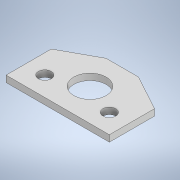
# Autodesk Inventor part: PositioningStop
Saved by Autodesk Inventor 2022.2 (Build 262287030, 287C)
## iProperties
Created: 2023-02-06
Part Number: PositioningStop
Material: Generic
Document SubType Name: Modeling
Designer: jak27277
Density: 1 g/cm^3
Appearance: Default
Author: jak27277
Autodesk Inventor part; units mm, degrees
ref_plane "YZ Plane" through (0, 0, 0) normal (1, 0, 0) x (0, 1, 0)
ref_plane "XZ Plane" through (0, 0, 0) normal (0, 1, 0) x (-1, 0, 0)
ref_plane "XY Plane" through (0, 0, 0) normal (0, 0, 1) x (1, 0, 0)
sketch "Sketch1" plane through (0, 0, 0) normal (0, 1, 0) x (-1, 0, 0)
  circle A0 centre (0, 0) radius 15.875
  line L0 (0, -31.75) -> (15.875, -31.75)
  line L1 (15.875, -31.75) -> (50.8, -12.7)
  line L2 (50.8, -12.7) -> (50.8, 31.75)
  line L3 (50.8, 31.75) -> (0, 31.75)
  circle A1 centre (31.75, 12.7) radius 6.35
  line L4 (0, -31.75) -> (0, 31.75)
  line L5 (0, -31.75) -> (-15.875, -31.75)
  line L6 (-15.875, -31.75) -> (-50.8, -12.7)
  line L7 (-50.8, -12.7) -> (-50.8, 31.75)
  line L8 (-50.8, 31.75) -> (0, 31.75)
  circle A2 centre (-31.75, 12.7) radius 6.35
  point P0 (0, 0)
  dimension "d6" = 101.6
  dimension "d7" = 19.05
  dimension "d8" = 19.05
  dimension "d9" = 31.75
  dimension "d10" = 31.75
  dimension "d11" = 63.5
  dimension "d12" = 44.45
  dimension "d13" = 12.7
  dimension "d14" = 31.75
  constraints: 18 end point, 4 symmetric about line, 3 centre point, 2 midpoint, 2 perpendicular, 1 horizontal, 1 vertical, 2 other
  measures "d6" distance between parallel lines of L7 L2
  measures "d7" distance from line of A2.centre L7
  measures "d8" distance from line of L8 A2.centre
  measures "d9" distance from line of A0.centre L8
  measures "d10" distance of L6.start L0.end
  measures "d11" distance between parallel lines of L0 L3
  measures "d12" distance of L7.start L8.start
  measures "d13" diameter of A2
  measures "d14" diameter of A0
extrude "Extrusion1" add sketch "Sketch1" along normal blind 6.35 contours A0 L4 L3 L2 L1 L0 | A0 L4 L5 L6 L7 L8
body "Solid1"
